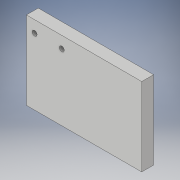
# Autodesk Inventor part: Kermit Bumper 2 Small
Saved by Autodesk Inventor 2018.2 (Build 222227000, 227)
## iProperties
Created: 2018-02-13
Part Number: Kermit Bumper 2 Small
Material: Generic
Document SubType Name: Modeling
Designer: kalra.rohan
Density: 1 g/cm^3
Appearance: Default
Author: kalra.rohan
Autodesk Inventor part; units mm, degrees
ref_plane "YZ Plane" through (0, 0, 0) normal (1, 0, 0) x (0, 1, 0)
ref_plane "XZ Plane" through (0, 0, 0) normal (0, 1, 0) x (-1, 0, 0)
ref_plane "XY Plane" through (0, 0, 0) normal (0, 0, 1) x (1, 0, 0)
sketch "Sketch1" plane through (0, 0, 0) normal (0, 0, 1) x (1, 0, 0)
  line L0 (0, 0) -> (177.8, 0)
  line L1 (177.8, 0) -> (177.8, -120.65)
  line L2 (177.8, -120.65) -> (0, -120.65)
  line L3 (0, -120.65) -> (0, 0)
  circle A0 centre (12.7, -18.0174) radius 3.81
  circle A1 centre (54.61, -18.0174) radius 3.81
  dimension "d0" = 120.65
  dimension "d1" = 177.8
  dimension "d2" = 7.62
  dimension "d3" = 12.7
  dimension "d4" = 7.62
  dimension "d5" = 41.91
  constraints: 8 end point, 2 centre point, 2 parallel, 1 horizontal, 1 perpendicular
  measures "d0" distance between parallel lines of L2 L0
  measures "d1" distance between parallel lines of L1 L3
  measures "d2" diameter of A0
  measures "d3" distance from line of A0.centre L3
  measures "d4" diameter of A1
  measures "d5" distance of A1.centre A0.centre
extrude "Extrusion1" add sketch "Sketch1" against normal blind 18.3261
body "Solid1"
